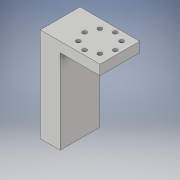
# Autodesk Inventor part: wheel arm stand off
Saved by Autodesk Inventor 2019 (Build 230136000, 136)
## iProperties
Created: 2019-10-26
Part Number: wheel arm stand off
Material: Generic
Document SubType Name: Modeling
Designer: User
Density: 1 g/cm^3
Appearance: Default
Author: User
Autodesk Inventor part; units mm, degrees
ref_plane "YZ Plane" through (0, 0, 0) normal (1, 0, 0) x (0, 1, 0)
ref_plane "XZ Plane" through (0, 0, 0) normal (0, 1, 0) x (-1, 0, 0)
ref_plane "XY Plane" through (0, 0, 0) normal (0, 0, 1) x (1, 0, 0)
sketch "Sketch4" plane through (0, 0, 0) normal (0, 0, 1) x (1, 0, 0)
  line L0 (0, 0) -> (0, 60.2234)
  line L1 (0, 60.2234) -> (25.4, 60.2234)
  line L2 (25.4, 60.2234) -> (25.4, 53.8734)
  line L3 (25.4, 53.8734) -> (0, 53.8734)
  line L4 (0, 60.2234) -> (-12.7, 60.2234)
  line L5 (-12.7, 60.2234) -> (-12.7, 0)
  line L6 (-12.7, 0) -> (0, 0)
  dimension "d25" = 60.2234
  dimension "d26" = 6.35
  dimension "d27" = 25.4
  dimension "d28" = 12.7
  constraints: 14 end point, 5 perpendicular, 1 horizontal, 1 point on line, 1 vertical
  measures "d25" distance of L0.start L0.end
  measures "d26" distance between parallel lines of L1 L3
  measures "d27" distance between parallel lines of L0 L2
  measures "d28" distance of L0.end L4.end
extrude "Extrusion3" add sketch "Sketch4" along normal blind 25.4
sketch "Sketch5" plane through (-12.7, 60.2234, 0) normal (0, 1, 0) x (1, 0, 0)
  circle A0 centre (25.4, -12.7) radius 9.779
  line L0 (38.1, 0) -> (38.1, -25.4) projected
  line L1 (38.1, 0) -> (0, 0) projected
  point P0 (12.7, 0)
  point P1 (15.621, -12.7)
  point P2 (18.4852, -19.6148)
  point P3 (25.4, -22.479)
  point P4 (32.3148, -19.6148)
  point P5 (35.179, -12.7)
  point P6 (32.3148, -5.7852)
  point P7 (25.4, -2.921)
  point P8 (18.4852, -5.7852)
  dimension "d31" = 19.558
  dimension "d32" = 12.7
  dimension "d33" = 12.7
  dimension "d36" = 360
  constraints: 1 horizontal alignment, 11 other
  measures "d32" distance from line of L0 point (25.4, -12.7)
  measures "d33" distance from line of L1 point (25.4, -12.7)
hole "Hole2" at (2.921, 60.2234, 12.7) at (5.7852, 60.2234, 19.6148) at (12.7, 60.2234, 22.479) at (19.6148, 60.2234, 19.6148) at (22.479, 60.2234, 12.7) at (19.6148, 60.2234, 5.7852) at (12.7, 60.2234, 2.921) at (5.7852, 60.2234, 5.7852) direction (0, -1, 0) diameter 2.7178 end through all
body "Solid3"
